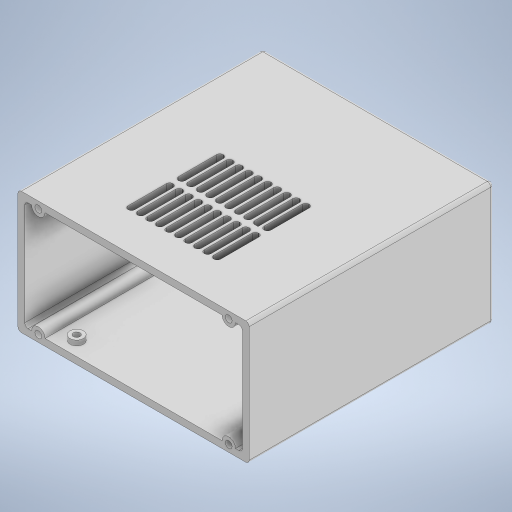
# Autodesk Inventor part: Case_Front
Saved by Autodesk Inventor 2023 (Build 270158000, 158)
## iProperties
Created: 2022-12-05
Part Number: Case_Front
Material: Generic
Document SubType Name: Modeling
Designer: elect
Density: 1 g/cm^3
Appearance: Default
Author: elect
Autodesk Inventor part; units mm, degrees
ref_plane "YZ Plane" through (0, 0, 0) normal (1, 0, 0) x (0, 1, 0)
ref_plane "XZ Plane" through (0, 0, 0) normal (0, 1, 0) x (-1, 0, 0)
ref_plane "XY Plane" through (0, 0, 0) normal (0, 0, 1) x (1, 0, 0)
sketch "Sketch1" plane through (0, 0, 0) normal (0, 0, 1) x (1, 0, 0)
  line L0 (1.5875, 0) -> (106.3625, 0)
  line L1 (107.95, 1.5875) -> (107.95, 55.5625)
  line L2 (106.3625, 57.15) -> (1.5875, 57.15)
  line L3 (0, 55.5625) -> (0, 1.5875)
  arc A0 (1.5875, 57.15) -> (0, 55.5625) centre (1.5875, 55.5625) ccw
  arc A1 (107.95, 55.5625) -> (106.3625, 57.15) centre (106.3625, 55.5625) ccw
  arc A2 (106.3625, 0) -> (107.95, 1.5875) centre (106.3625, 1.5875) ccw
  arc A3 (0, 1.5875) -> (1.5875, 0) centre (1.5875, 1.5875) ccw
  point P0 (0, 0)
  point P1 (107.95, 57.15)
  point P2 (0, 57.15)
  dimension "d0" = 107.95
  dimension "d1" = 57.15
  dimension "d2" = 1.5875
  dimension "d3" = 1.5875
  constraints: 8 end point, 8 point on circle, 8 tangent, 6 point on line, 4 centre point, 2 equal radius, 2 parallel, 1 horizontal, 1 perpendicular
  measures "d0" distance of point (107.95, 57.15) point (0, 57.15)
  measures "d1" distance of point (0, 57.15) point (0, 0)
  measures "d2" radius of A0
  measures "d3" radius of A1
extrude "Extrusion1" add sketch "Sketch1" along normal blind 114.3
sketch "Sketch2" plane through (0, 0, 114.3) normal (0, 0, 1) x (1, 0, 0)
  line L0 (104.775, 52.3875) -> (104.775, 4.7625)
  line L1 (3.175, 4.7625) -> (3.175, 52.3875)
  arc A0 (4.7625, 53.975) -> (3.175, 52.3875) centre (4.7625, 52.3875) ccw
  arc A1 (104.775, 52.3875) -> (103.1875, 53.975) centre (103.1875, 52.3875) ccw
  arc A2 (103.1875, 3.175) -> (104.775, 4.7625) centre (103.1875, 4.7625) ccw
  arc A3 (3.175, 4.7625) -> (4.7625, 3.175) centre (4.7625, 4.7625) ccw
  line L2 (106.3625, 57.15) -> (1.5875, 57.15) projected
  line L3 (0, 55.5625) -> (0, 1.5875) projected
  line L4 (1.5875, 0) -> (106.3625, 0) projected
  line L5 (107.95, 1.5875) -> (107.95, 55.5625) projected
  line L6 (4.7625, 53.975) -> (6.35, 53.975)
  line L7 (12.7, 53.975) -> (95.25, 53.975)
  line L8 (101.6, 53.975) -> (103.1875, 53.975)
  line L9 (103.1875, 3.175) -> (101.6, 3.175)
  line L10 (95.25, 3.175) -> (12.7, 3.175)
  line L11 (6.35, 3.175) -> (4.7625, 3.175)
  arc A4 (6.35, 53.975) -> (12.7, 53.975) centre (9.525, 53.975) ccw
  arc A5 (95.25, 53.975) -> (101.6, 53.975) centre (98.425, 53.975) ccw
  arc A6 (12.7, 3.175) -> (6.35, 3.175) centre (9.525, 3.175) ccw
  arc A7 (101.6, 3.175) -> (95.25, 3.175) centre (98.425, 3.175) ccw
  point P0 (0, 0)
  point P1 (100.0125, 53.975)
  point P2 (11.1125, 53.975)
  dimension "d6" = 1.5875
  dimension "d8" = 3.175
  dimension "d10" = 3.175
  dimension "d73" = 3.175
  dimension "d75" = 6.35
  dimension "d76" = 6.35
  dimension "d77" = 6.35
  constraints: 16 end point, 16 point on circle, 16 tangent, 10 parallel, 8 centre point, 6 equal radius, 4 point on line, 3 horizontal, 3 perpendicular, 2 vertical alignment
  measures "d6" radius of A0
  measures "d8" distance between parallel lines of L1 L3
  measures "d10" distance between parallel lines of L5 L0
  measures "d73" distance between parallel lines of L2 L7
  measures "d75" distance from line of L1 A4.centre
  measures "d76" distance from line of L0 A5.centre
  measures "d77" diameter of A4
extrude "Extrusion2" cut sketch "Sketch2" against normal blind 111.125
fillet "Fillet1" radius 1.5875 8 edges at (0.465, 56.685, 0) (0, 28.575, 0) (0.465, 0.465, 0) (53.975, 0, 0) (107.485, 0.465, 0) (107.95, 28.575, 0) (107.485, 56.685, 0) (53.975, 57.15, 0)
sketch "Sketch3" plane through (0, 0, 0) normal (0, 0, -1) x (-1, 0, 0)
  line L0 (-82.8675, 44.5135) -> (-25.0825, 44.5135)
  line L1 (-23.495, 42.926) -> (-23.495, 20.701)
  line L2 (-25.0825, 19.1135) -> (-82.8675, 19.1135)
  line L3 (-84.455, 20.701) -> (-84.455, 42.926)
  line L4 (-1.5875, 1.5875) -> (-106.3625, 1.5875) projected
  line L5 (-106.3625, 55.5625) -> (-1.5875, 55.5625) projected
  line L6 (-1.5875, 55.5625) -> (-1.5875, 1.5875) projected
  line L7 (-106.3625, 1.5875) -> (-106.3625, 55.5625) projected
  arc A0 (-82.8675, 44.5135) -> (-84.455, 42.926) centre (-82.8675, 42.926) ccw
  arc A1 (-84.455, 20.701) -> (-82.8675, 19.1135) centre (-82.8675, 20.701) ccw
  arc A2 (-25.0825, 19.1135) -> (-23.495, 20.701) centre (-25.0825, 20.701) ccw
  arc A3 (-23.495, 42.926) -> (-25.0825, 44.5135) centre (-25.0825, 42.926) ccw
  point P0 (0, 0)
  point P1 (-84.455, 44.5135)
  point P2 (-23.495, 44.5135)
  point P3 (-84.455, 19.1135)
  point P4 (-23.495, 31.8135)
  dimension "d17" = 60.96
  dimension "d18" = 25.4
  dimension "d19" = 17.526
  dimension "d20" = 11.049
  dimension "d21" = 21.9075
  dimension "d22" = 21.9075
  dimension "d23" = 1.5875
  constraints: 8 end point, 8 point on circle, 8 tangent, 6 point on line, 4 centre point, 3 equal radius, 2 parallel, 1 horizontal, 1 midpoint, 1 perpendicular
  measures "d17" distance of point (-84.455, 44.513) point (-23.495, 44.514)
  measures "d18" distance of point (-84.455, 19.113) point (-84.455, 44.513)
  measures "d19" distance between parallel lines of L4 L2
  measures "d20" distance between parallel lines of L5 L0
  measures "d21" distance from line of L6 point (-23.495, 31.814)
  measures "d22" distance between parallel lines of L7 L3
  measures "d23" radius of A0
extrude "Extrusion3" cut sketch "Sketch3" against normal blind 111.125 contours L0 A3 L1 A2 L2 A1 L3 A0
fillet "Fillet2" radius 1.5875 8 edges at (23.96, 44.0485, 0) (23.495, 31.8135, 0) (23.96, 19.5785, 0) (53.975, 19.1135, 0) (83.99, 19.5785, 0) (84.455, 31.8135, 0) (83.99, 44.0485, 0) (53.975, 44.5135, 0)
sketch "Sketch4" plane through (0, 0, 3.175) normal (0, 0, 1) x (1, 0, 0)
  line L0 (20.955, 47.6885) -> (86.995, 47.6885)
  line L1 (86.995, 47.6885) -> (86.995, 15.9385)
  line L2 (86.995, 15.9385) -> (20.955, 15.9385)
  line L3 (20.955, 15.9385) -> (20.955, 47.6885)
  line L4 (25.0825, 19.1135) -> (82.8675, 19.1135) projected
  line L5 (82.8675, 44.5135) -> (25.0825, 44.5135) projected
  line L6 (23.495, 42.926) -> (23.495, 20.701) projected
  line L7 (84.455, 20.701) -> (84.455, 42.926) projected
  line L8 (43.815, 47.6885) -> (64.135, 47.6885)
  line L9 (64.135, 47.6885) -> (64.135, 50.2285)
  line L10 (64.135, 50.2285) -> (43.815, 50.2285)
  line L11 (43.815, 50.2285) -> (43.815, 47.6885)
  line L12 (86.995, 40.0685) -> (89.535, 40.0685)
  line L13 (89.535, 40.0685) -> (89.535, 23.5585)
  line L14 (89.535, 23.5585) -> (86.995, 23.5585)
  line L15 (86.995, 23.5585) -> (86.995, 40.0685)
  line L16 (43.815, 15.9385) -> (64.135, 15.9385)
  line L17 (64.135, 15.9385) -> (64.135, 13.3985)
  line L18 (64.135, 13.3985) -> (43.815, 13.3985)
  line L19 (43.815, 13.3985) -> (43.815, 15.9385)
  line L20 (20.955, 40.0685) -> (18.415, 40.0685)
  line L21 (18.415, 40.0685) -> (18.415, 23.5585)
  line L22 (18.415, 23.5585) -> (20.955, 23.5585)
  line L23 (20.955, 23.5585) -> (20.955, 40.0685)
  circle A0 centre (12.7, 44.5135) radius 2.54
  circle A1 centre (94.5614, 44.5135) radius 2.54
  circle A2 centre (12.446, 37.1519) radius 2.667
  circle A3 centre (12.446, 28.1095) radius 2.667
  circle A4 centre (12.446, 19.0671) radius 2.667
  circle A5 centre (94.361, 37.1502) radius 2.667
  circle A6 centre (94.361, 28.1078) radius 2.667
  circle A7 centre (94.361, 19.0654) radius 1.5875
  point P0 (0, 0)
  point P1 (19.685, 40.0685)
  point P2 (19.685, 23.5585)
  point P3 (43.815, 48.9585)
  point P4 (64.135, 15.9385)
  point P5 (64.135, 47.6885)
  dimension "d27" = 66.04
  dimension "d28" = 31.75
  dimension "d29" = 3.175
  dimension "d30" = 3.175
  dimension "d31" = 2.54
  dimension "d32" = 2.54
  dimension "d33" = 7.62
  dimension "d34" = 7.62
  dimension "d35" = 2.54
  dimension "d36" = 7.62
  dimension "d37" = 7.62
  dimension "d38" = 2.54
  dimension "d39" = 22.86
  dimension "d40" = 22.86
  dimension "d41" = 2.54
  dimension "d42" = 22.86
  dimension "d43" = 22.86
  dimension "d44" = 2.54
  dimension "d47" = 81.8614
  dimension "d48" = 0
  dimension "d49" = 10.795
  dimension "d50" = 5.08
  dimension "d78" = 5.334
  dimension "d79" = 7.366
  dimension "d80" = 7.366
  dimension "d81" = 9.0424
  dimension "d82" = 9.0424
  dimension "d83" = 9.0424
  dimension "d84" = 9.0424
  dimension "d87" = 3.175
  dimension "d104" = 11.049
  dimension "d105" = 9.906
  constraints: 40 end point, 10 parallel, 8 centre point, 5 equal radius, 5 horizontal, 5 perpendicular, 4 point on line, 4 vertical alignment, 3 midpoint, 1 horizontal alignment
  measures "d27" distance of L0.start L0.end
  measures "d28" distance of L2.end L0.start
  measures "d29" distance between parallel lines of L4 L2
  measures "d30" distance between parallel lines of L5 L0
  measures "d31" distance between parallel lines of L6 L3
  measures "d32" distance between parallel lines of L1 L7
  measures "d33" distance from line of point (19.685, 40.069) L0
  measures "d34" distance from line of L2 point (19.685, 23.558)
  measures "d35" distance between parallel lines of L3 L21
  measures "d36" distance between parallel lines of L2 L14
  measures "d37" distance between parallel lines of L0 L12
  measures "d38" distance between parallel lines of L1 L13
  measures "d39" distance between parallel lines of L1 L9
  measures "d40" distance from line of L3 point (43.815, 48.958)
  measures "d41" distance between parallel lines of L8 L10
  measures "d42" distance between parallel lines of L1 L17
  measures "d43" distance between parallel lines of L3 L19
  measures "d44" distance between parallel lines of L16 L18
  measures "d47" distance of A1.centre A0.centre
  measures "d48" distance from line of L5 A0.centre
  measures "d49" distance from line of L6 A0.centre
  measures "d50" diameter of A0
  measures "d78" diameter of A2
  measures "d79" distance of A0.centre A2.centre
  measures "d80" distance of A1.centre A5.centre
  measures "d81" distance of A3.centre A2.centre
  measures "d82" distance of A4.centre A3.centre
  measures "d83" distance of A6.centre A5.centre
  measures "d84" distance of A6.centre A7.centre
  measures "d87" diameter of A7
  measures "d104" distance from line of L6 A2.centre
  measures "d105" distance from line of L7 A5.centre
extrude "Extrusion4" add sketch "Sketch4" along normal blind 3.175 contours L11 L10 L9 L0 | L3 L22 L21 L20 | L12 L13 L14 L1 | L2 L17 L18 L19
extrude "Extrusion5" cut sketch "Sketch4" against normal blind 25.4 contours A2 | A3 | A4 | A5 | A6 | A7
extrude "Extrusion6" add sketch "Sketch4" along normal blind 12.7 contours A0 | A1
hole "Hole4" at (12.7, 44.5135, 3.175) at (94.5614, 44.5135, 3.175) direction (0, 0, 1) diameter 3.175 end through all
hole "Hole5" at (9.525, 53.975, 114.3) at (98.425, 53.975, 114.3) at (98.425, 3.175, 114.3) at (9.525, 3.175, 114.3) direction (0, 0, -1) diameter 3.175 depth 50.8 tip angle 118
sketch "Sketch5" plane through (12.7, 3.175, 114.3) normal (0, 1, 0) x (1, 0, 0)
  circle A0 centre (8.128, 6.604) radius 3.175
  line L0 (-11.1125, 0) -> (93.6625, 0) projected
  line L1 (-12.7, 112.7125) -> (-12.7, 0) projected
  point P0 (-12.7, 114.3)
  dimension "d106" = 6.35
  dimension "d107" = 6.604
  dimension "d108" = 20.828
  constraints: 1 centre point
  measures "d106" diameter of A0
  measures "d107" distance from line of L0 A0.centre
  measures "d108" distance from line of L1 A0.centre
extrude "Extrusion7" add sketch "Sketch5" along normal blind 2.286
sketch "Sketch6" plane through (20.828, 5.461, 107.696) normal (0, 1, 0) x (1, 0, 0)
  circle A0 centre (0, 0) radius 3.175 projected
  point P0 (-20.828, 107.696)
  constraints: 1 coincident
hole "Hole6" at (20.828, 5.461, 107.696) direction (0, -1, 0) diameter 3.175 depth 3.175 tip angle 118
sketch "Sketch7" plane through (0, 0, 0) normal (0, 0, -1) x (-1, 0, 0)
  line L0 (-84.7724, 13.1636) -> (-21.2726, 13.0175) construction
  line L1 (-21.2726, 13.0175) -> (-21.3018, 0.3175) construction
  line L2 (-21.3018, 0.3175) -> (-84.8016, 0.4636) construction
  line L3 (-84.8016, 0.4636) -> (-84.7724, 13.1636) construction
  line L4 (-106.3625, 1.5875) -> (-106.3625, 55.5625) projected
  line L5 (-1.5875, 1.5875) -> (-106.3625, 1.5875) projected
  line L6 (-106.3625, 55.5625) -> (-1.5875, 55.5625)
  line L7 (-1.5875, 55.5625) -> (-1.5875, 1.5875)
  line L8 (-100.711, 43.307) -> (-88.011, 43.307) construction
  line L9 (-88.011, 43.307) -> (-88.011, 40.132) construction
  line L10 (-88.011, 40.132) -> (-100.711, 40.132) construction
  line L11 (-100.711, 40.132) -> (-100.711, 43.307) construction
  line L12 (-100.711, 34.163) -> (-88.011, 34.163) construction
  line L13 (-88.011, 34.163) -> (-88.011, 30.988) construction
  line L14 (-88.011, 30.988) -> (-100.711, 30.988) construction
  line L15 (-100.711, 30.988) -> (-100.711, 34.163) construction
  line L16 (-100.711, 25.273) -> (-88.011, 25.273) construction
  line L17 (-88.011, 25.273) -> (-88.011, 22.098) construction
  line L18 (-88.011, 22.098) -> (-100.711, 22.098) construction
  line L19 (-100.711, 22.098) -> (-100.711, 25.273) construction
  line L20 (-82.8675, 17.526) -> (-25.0825, 17.526) projected
  circle A0 centre (-94.361, 37.1502) radius 2.667 projected
  line L21 (-21.336, 43.307) -> (-3.556, 43.307) construction
  line L22 (-3.556, 43.307) -> (-3.556, 40.132) construction
  line L23 (-3.556, 40.132) -> (-21.336, 40.132) construction
  line L24 (-21.336, 40.132) -> (-21.336, 43.307) construction
  line L25 (-21.336, 34.163) -> (-3.556, 34.163) construction
  line L26 (-3.556, 34.163) -> (-3.556, 30.988) construction
  line L27 (-3.556, 30.988) -> (-21.336, 30.988) construction
  line L28 (-21.336, 30.988) -> (-21.336, 34.163) construction
  line L29 (-21.336, 25.273) -> (-3.556, 25.273) construction
  line L30 (-3.556, 25.273) -> (-3.556, 22.098) construction
  line L31 (-3.556, 22.098) -> (-21.336, 22.098) construction
  line L32 (-21.336, 22.098) -> (-21.336, 25.273) construction
  circle A1 centre (-12.446, 37.1519) radius 2.667 projected
  line L33 (-59.3387, 12.9994) -> (-57.4495, 12.9951)
  line L34 (-57.4495, 12.9951) -> (-57.4571, 9.6802)
  spline S0 degree 2 poles (-57.4571, 9.6802) (-57.4595, 8.6417) (-57.8317, 7.5512) (-58.954, 6.7969) (-59.8224, 6.7989) knots 0 0 0 1 2 3 3 3
  spline S1 degree 2 poles (-59.8224, 6.7989) (-60.7435, 6.8011) (-61.7574, 7.3021) (-62.3067, 8.2656) (-62.3579, 8.9698) knots 0 0 0 1 2 3 3 3
  line L35 (-62.3579, 8.9698) -> (-60.5561, 9.212)
  spline S2 degree 2 poles (-60.5561, 9.212) (-60.5512, 8.8072) (-60.423, 8.4197) (-60.2648, 8.2961) knots 0 0 0 1 2 2 2
  spline S3 degree 2 poles (-60.2648, 8.2961) (-60.1594, 8.2196) (-59.9599, 8.2191) knots 0 0 0 1 1 1
  spline S4 degree 2 poles (-59.9599, 8.2191) (-59.6431, 8.2184) (-59.3487, 8.6871) (-59.3474, 9.2445) knots 0 0 0 1 2 2 2
  line L36 (-59.3474, 9.2445) -> (-59.3387, 12.9994)
  line L37 (-56.1587, 12.9921) -> (-53.3601, 12.9857)
  spline S5 degree 2 poles (-53.3601, 12.9857) (-52.5328, 12.9838) (-51.513, 12.5297) (-50.8519, 11.6891) (-50.5553, 10.5737) (-50.5567, 9.9518) knots 0 0 0 1 2 3 4 4 4
  spline S6 degree 2 poles (-50.5567, 9.9518) (-50.559, 8.972) (-51.0073, 7.8993) (-51.7952, 7.1736) (-52.2531, 7.0514) knots 0 0 0 1 2 3 3 3
  spline S7 degree 2 poles (-52.2531, 7.0514) (-52.8696, 6.8885) (-53.3741, 6.8897) knots 0 0 0 1 1 1
  line L38 (-53.3741, 6.8897) -> (-56.1728, 6.8961)
  line L39 (-56.1728, 6.8961) -> (-56.1587, 12.9921)
  line L40 (-54.2786, 11.609) -> (-54.2862, 8.2765)
  line L41 (-54.2862, 8.2765) -> (-53.8227, 8.2754)
  spline S8 degree 2 poles (-53.8227, 8.2754) (-53.236, 8.2741) (-52.7367, 8.5369) (-52.4536, 9.1875) (-52.4519, 9.9209) knots 0 0 0 1 2 3 3 3
  spline S9 degree 2 poles (-52.4519, 9.9209) (-52.4496, 10.889) (-53.0817, 11.6063) (-53.8092, 11.6079) knots 0 0 0 1 2 2 2
  line L42 (-53.8092, 11.6079) -> (-54.2786, 11.609)
  line L43 (-45.5064, 9.3652) -> (-43.8589, 8.8627)
  spline S10 degree 2 poles (-43.8589, 8.8627) (-44.0247, 8.1707) (-44.7427, 7.2395) (-45.8057, 6.7667) (-46.6213, 6.7686) knots 0 0 0 1 2 3 3 3
  spline S11 degree 2 poles (-46.6213, 6.7686) (-47.6187, 6.7709) (-48.8729, 7.3546) (-49.7849, 8.8118) (-49.7822, 9.9441) knots 0 0 0 1 2 3 3 3
  spline S12 degree 2 poles (-49.7822, 9.9441) (-49.7788, 11.4579) (-48.1674, 13.0794) (-46.6948, 13.076) knots 0 0 0 1 2 2 2
  spline S13 degree 2 poles (-46.6948, 13.076) (-45.5448, 13.0733) (-44.2327, 12.1374) (-43.9122, 11.1745) knots 0 0 0 1 2 2 2
  line L44 (-43.9122, 11.1745) -> (-45.5793, 10.8087)
  spline S14 degree 2 poles (-45.5793, 10.8087) (-45.6667, 11.0846) (-45.7603, 11.2139) knots 0 0 0 1 1 1
  spline S15 degree 2 poles (-45.7603, 11.2139) (-45.9182, 11.4314) (-46.3753, 11.6671) (-46.6569, 11.6678) knots 0 0 0 1 2 2 2
  spline S16 degree 2 poles (-46.6569, 11.6678) (-47.2906, 11.6692) (-47.6321, 11.1537) knots 0 0 0 1 1 1
  spline S17 degree 2 poles (-47.6321, 11.1537) (-47.8911, 10.7729) (-47.893, 9.9515) knots 0 0 0 1 1 1
  spline S18 degree 2 poles (-47.893, 9.9515) (-47.8953, 8.9365) (-47.281, 8.1841) (-46.7236, 8.1828) knots 0 0 0 1 2 2 2
  spline S19 degree 2 poles (-46.7236, 8.1828) (-46.1838, 8.1816) (-45.6309, 8.7846) (-45.5064, 9.3652) knots 0 0 0 1 2 2 2
  point P0 (0, 0)
  point P1 (-53.0225, 13.0905)
  point P2 (-21.2872, 6.6675)
  point P3 (-94.361, 43.307)
  point P4 (-94.361, 34.163)
  point P5 (-94.361, 25.273)
  point P6 (-100.711, 23.6855)
  point P7 (-12.446, 43.307)
  point P8 (-12.446, 34.163)
  point P9 (-12.446, 25.273)
  point P10 (-88.011, 41.7195)
  point P11 (-21.336, 41.7195)
  point P12 (-21.336, 32.5755)
  point P13 (-88.011, 32.5755)
  point P14 (-88.011, 23.6855)
  point P15 (-21.336, 23.6855)
  dimension "d118" = 53.34
  dimension "d119" = 5.08
  dimension "d120" = 12.7
  dimension "d121" = 63.5
  dimension "d124" = 12.7
  dimension "d125" = 12.7
  dimension "d126" = 12.7
  dimension "d127" = 3.175
  dimension "d128" = 3.175
  dimension "d129" = 3.175
  dimension "d134" = 17.78
  dimension "d135" = 17.78
  dimension "d136" = 17.78
  dimension "d137" = 3.175
  dimension "d138" = 3.175
  dimension "d139" = 3.175
  dimension "d140" = 4.572
  dimension "d141" = 13.462
  dimension "d142" = 22.606
  constraints: 15 midpoint, 6 vertical alignment, 4 end point, 3 horizontal alignment, 2 coincident, 1 horizontal, 1 perpendicular, 14 other
  measures "d118" distance from line of L4 point (-53.022, 13.091)
  measures "d119" distance from line of L5 point (-21.287, 6.668)
  measures "d120" distance between parallel lines of L2 L0
  measures "d121" distance of L0.start L0.end
  measures "d124" distance of L16.start L16.end
  measures "d125" distance of L12.start L12.end
  measures "d126" distance of L8.start L8.end
  measures "d127" distance of L8.end L9.end
  measures "d128" distance of L12.end L13.end
  measures "d129" distance of L16.end L17.end
  measures "d134" distance of L21.start L21.end
  measures "d135" distance of L25.start L25.end
  measures "d136" distance of L29.start L29.end
  measures "d137" distance of L21.end L22.end
  measures "d138" distance of L25.end L26.end
  measures "d139" distance of L29.end L30.end
  measures "d140" distance between parallel lines of L20 L31
  measures "d141" distance between parallel lines of L20 L27
  measures "d142" distance between parallel lines of L20 L23
sketch "Sketch8" plane through (1.5875, 57.15, 114.3) normal (0, 1, 0) x (1, 0, 0)
  line L0 (30.7975, 61.9125) -> (33.9725, 61.9125)
  line L1 (33.9725, 61.9125) -> (33.9725, 17.4625)
  line L2 (33.9725, 17.4625) -> (30.7975, 17.4625)
  line L3 (30.7975, 17.4625) -> (30.7975, 61.9125)
  line L4 (0, 112.7125) -> (0, 0) projected
  line L5 (0, 103.6948) -> (98.6325, 103.6948)
  line L6 (100.0125, 0) -> (100.0125, 111.125) projected
  line L7 (38.4175, 61.9125) -> (38.4175, 17.4625)
  line L8 (35.2425, 17.4625) -> (35.2425, 61.9125)
  line L9 (35.2425, 61.9125) -> (38.4175, 61.9125)
  line L10 (38.4175, 17.4625) -> (35.2425, 17.4625)
  line L11 (42.8625, 61.9125) -> (42.8625, 17.4625)
  line L12 (39.6875, 17.4625) -> (39.6875, 61.9125)
  line L13 (39.6875, 61.9125) -> (42.8625, 61.9125)
  line L14 (42.8625, 17.4625) -> (39.6875, 17.4625)
  line L15 (47.3075, 61.9125) -> (47.3075, 17.4625)
  line L16 (44.1325, 17.4625) -> (44.1325, 61.9125)
  line L17 (44.1325, 61.9125) -> (47.3075, 61.9125)
  line L18 (47.3075, 17.4625) -> (44.1325, 17.4625)
  line L19 (51.7525, 61.9125) -> (51.7525, 17.4625)
  line L20 (48.5775, 17.4625) -> (48.5775, 61.9125)
  line L21 (48.5775, 61.9125) -> (51.7525, 61.9125)
  line L22 (51.7525, 17.4625) -> (48.5775, 17.4625)
  line L23 (56.1975, 61.9125) -> (56.1975, 17.4625)
  line L24 (53.0225, 17.4625) -> (53.0225, 61.9125)
  line L25 (53.0225, 61.9125) -> (56.1975, 61.9125)
  line L26 (56.1975, 17.4625) -> (53.0225, 17.4625)
  line L27 (60.6425, 61.9125) -> (60.6425, 17.4625)
  line L28 (57.4675, 17.4625) -> (57.4675, 61.9125)
  line L29 (57.4675, 61.9125) -> (60.6425, 61.9125)
  line L30 (60.6425, 17.4625) -> (57.4675, 17.4625)
  line L31 (65.0875, 61.9125) -> (65.0875, 17.4625)
  line L32 (61.9125, 17.4625) -> (61.9125, 61.9125)
  line L33 (61.9125, 61.9125) -> (65.0875, 61.9125)
  line L34 (65.0875, 17.4625) -> (61.9125, 17.4625)
  line L35 (69.5325, 61.9125) -> (69.5325, 17.4625)
  line L36 (66.3575, 17.4625) -> (66.3575, 61.9125)
  line L37 (66.3575, 61.9125) -> (69.5325, 61.9125)
  line L38 (69.5325, 17.4625) -> (66.3575, 17.4625)
  line L39 (73.9775, 61.9125) -> (73.9775, 17.4625)
  line L40 (70.8025, 17.4625) -> (70.8025, 61.9125)
  line L41 (70.8025, 61.9125) -> (73.9775, 61.9125)
  line L42 (73.9775, 17.4625) -> (70.8025, 17.4625)
  line L43 (104.775, 112.7125) -> (104.775, 0) projected
  line L44 (0, 112.7125) -> (104.775, 112.7125) projected
  line L45 (30.7975, 40.9575) -> (33.9725, 40.9575)
  line L46 (30.7975, 38.4175) -> (33.9725, 38.4175)
  line L47 (35.2425, 38.4175) -> (38.4175, 38.4175)
  line L48 (35.2425, 40.9575) -> (38.4175, 40.9575)
  line L49 (39.6875, 40.9575) -> (42.8625, 40.9575)
  line L50 (39.6875, 38.4175) -> (42.8625, 38.4175)
  line L51 (44.1325, 40.9575) -> (47.3075, 40.9575)
  line L52 (44.1325, 38.4175) -> (47.3075, 38.4175)
  line L53 (48.5775, 40.9575) -> (51.7525, 40.9575)
  line L54 (48.5775, 38.4175) -> (51.7525, 38.4175)
  line L55 (53.0225, 40.9575) -> (56.1975, 40.9575)
  line L56 (53.0225, 38.4175) -> (56.1975, 38.4175)
  line L57 (57.4675, 40.9575) -> (60.6425, 40.9575)
  line L58 (57.4675, 38.4175) -> (60.6425, 38.4175)
  line L59 (61.9125, 40.9575) -> (65.0875, 40.9575)
  line L60 (61.9125, 38.4175) -> (65.0875, 38.4175)
  line L61 (66.3575, 40.9575) -> (69.5325, 40.9575)
  line L62 (70.8025, 40.9575) -> (73.9775, 40.9575)
  line L63 (66.3575, 38.4175) -> (69.5325, 38.4175)
  line L64 (70.8025, 38.4175) -> (73.9775, 38.4175)
  line L65 (30.7975, 40.9575) -> (30.7975, 38.4175)
  line L66 (33.9725, 38.4175) -> (33.9725, 40.9575)
  line L67 (35.2425, 40.9575) -> (35.2425, 38.4175)
  line L68 (38.4175, 40.9575) -> (38.4175, 38.4175)
  line L69 (39.6875, 40.9575) -> (39.6875, 38.4175)
  line L70 (42.8625, 40.9575) -> (42.8625, 38.4175)
  line L71 (44.1325, 40.9575) -> (44.1325, 38.4175)
  line L72 (47.3075, 38.4175) -> (47.3075, 40.9575)
  line L73 (48.5775, 40.9575) -> (48.5775, 38.4175)
  line L74 (51.7525, 40.9575) -> (51.7525, 38.4175)
  line L75 (53.0225, 40.9575) -> (53.0225, 38.4175)
  line L76 (56.1975, 40.9575) -> (56.1975, 38.4175)
  line L77 (57.4675, 40.9575) -> (57.4675, 38.4175)
  line L78 (60.6425, 40.9575) -> (60.6425, 38.4175)
  line L79 (61.9125, 40.9575) -> (61.9125, 38.4175)
  line L80 (65.0875, 40.9575) -> (65.0875, 38.4175)
  line L81 (66.3575, 38.4175) -> (66.3575, 40.9575)
  line L82 (69.5325, 40.9575) -> (69.5325, 38.4175)
  line L83 (70.8025, 40.9575) -> (70.8025, 38.4175)
  line L84 (73.9775, 40.9575) -> (73.9775, 38.4175)
  point P0 (-1.5875, 114.3)
  dimension "d143" = 3.175
  dimension "d144" = 44.45
  dimension "d147" = 4.445
  dimension "d152" = 30.7975
  dimension "d153" = 30.7975
  dimension "d154" = 50.8
  constraints: 162 end point, 41 point on line, 25 perpendicular, 14 collinear, 5 parallel, 2 horizontal, 72 other
  measures "d143" distance of L1.end L2.end
  measures "d144" distance of L2.end L0.start
  measures "d147" distance of L0.end L7.start
  measures "d152" distance between parallel lines of L4 L3
  measures "d153" distance between parallel lines of L43 L39
  measures "d154" distance between parallel lines of L0 L44
extrude "Extrusion8" cut sketch "Sketch8" against normal blind 25.4 contours L0 L1 L45 L3 | L46 L1 L2 L3 | L7 L48 L8 L9 | L7 L10 L8 L47 | L11 L49 L12 L13 | L11 L14 L12 L50 | L15 L51 L16 L17 | L15 L18 L16 L52 | L19 L53 L20 L21 | L19 L22 L20 L54 | L23 L55 L24 L25 | L23 L26 L24 L56 | L27 L57 L28 L29 | L27 L30 L28 L58 | L31 L59 L32 L33 | L31 L34 L32 L60 | L35 L61 L36 L37 | L35 L38 L36 L63 | L39 L62 L40 L41 | L39 L42 L40 L64
sketch "Sketch9" plane through (12.7, 53.975, 114.3) normal (0, -1, 0) x (1, 0, 0)
  line L0 (14.2875, -63.7812) -> (68.2625, -63.7812)
  line L1 (68.2625, -63.7812) -> (68.2625, -66.9562)
  line L2 (68.2625, -66.9562) -> (14.2875, -66.9562)
  line L3 (14.2875, -66.9562) -> (14.2875, -63.7812)
  line L4 (68.2625, -63.7812) -> (65.0875, -63.7812)
  line L5 (65.0875, -63.7812) -> (65.0875, -12.9812)
  line L6 (65.0875, -12.9812) -> (68.2625, -12.9812)
  line L7 (68.2625, -12.9812) -> (68.2625, -63.7812)
  line L8 (19.685, -17.4625) -> (19.685, -61.9125) projected
  line L9 (14.2875, -63.7812) -> (17.4625, -63.7812)
  line L10 (17.4625, -63.7812) -> (17.4625, -12.9812)
  line L11 (17.4625, -12.9812) -> (14.2875, -12.9812)
  line L12 (14.2875, -12.9812) -> (14.2875, -63.7812)
  line L13 (62.865, -61.9125) -> (62.865, -17.4625) projected
  point P0 (-12.7, -114.3)
  dimension "d157" = 53.975
  dimension "d158" = 3.175
  dimension "d159" = 3.175
  dimension "d160" = 5.3975
  dimension "d161" = 50.8
  dimension "d162" = 50.8
  dimension "d163" = 3.175
  dimension "d164" = 5.3975
  dimension "d165" = 47.625
  constraints: 24 end point, 6 parallel, 3 horizontal, 3 perpendicular
  measures "d157" distance of L1.end L2.end
  measures "d158" distance of L0.end L1.end
  measures "d159" distance between parallel lines of L7 L5
  measures "d160" distance between parallel lines of L8 L3
  measures "d161" distance of L11.end L0.start
  measures "d162" distance of L6.end L0.end
  measures "d163" distance between parallel lines of L10 L12
  measures "d164" distance between parallel lines of L13 L7
  measures "d165" distance between parallel lines of L5 L10
extrude "Extrusion9" add sketch "Sketch9" along normal blind 3.175
sketch "Sketch10" plane through (12.7, 50.8, 114.3) normal (0, -1, 0) x (1, 0, 0)
  line L0 (14.2875, -66.9562) -> (14.2875, -12.9812) projected
  line L1 (68.2625, -66.9562) -> (14.2875, -66.9562) projected
  line L2 (14.2875, -12.9812) -> (20.6375, -12.9812)
  line L3 (20.6375, -12.9812) -> (20.6375, -66.9562)
  line L4 (20.6375, -66.9562) -> (14.2875, -66.9562)
  line L5 (14.2875, -66.9562) -> (14.2875, -12.9812)
  line L6 (68.2625, -12.9812) -> (61.9125, -12.9812)
  line L7 (61.9125, -12.9812) -> (61.9125, -66.9562)
  line L8 (61.9125, -66.9562) -> (68.2625, -66.9562)
  line L9 (68.2625, -66.9562) -> (68.2625, -12.9812)
  line L10 (68.2625, -12.9812) -> (68.2625, -66.9562) projected
  line L11 (20.6375, -66.9562) -> (61.9125, -66.9562)
  line L12 (61.9125, -66.9562) -> (61.9125, -60.6062)
  line L13 (61.9125, -60.6062) -> (20.6375, -60.6062)
  line L14 (20.6375, -60.6062) -> (20.6375, -66.9562)
  point P0 (-12.7, -114.3)
  point P1 (41.275, -66.9562)
  point P2 (20.6375, -60.6062)
  dimension "d168" = 6.35
  dimension "d169" = 6.35
  dimension "d170" = 0
  dimension "d171" = 6.35
  constraints: 24 end point, 6 parallel, 4 point on line, 3 horizontal, 3 perpendicular, 1 midpoint
  measures "d168" distance of L0.end L2.end
  measures "d169" distance of L6.start L6.end
  measures "d170" distance between parallel lines of L10 L9
  measures "d171" distance from line of point (41.275, -66.956) L13
extrude "Extrusion10" add sketch "Sketch10" along normal blind 1.5875
chamfer "Chamfer2" distance 3.81 angle 50 1 edges at (53.975, 49.2125, 47.3438) measured on face at (53.975, 49.2125, 47.8438)
fillet "Fillet3" radius 3.175 2 edges at (26.9875, 49.2125, 76.2363) (80.9625, 49.2125, 76.2363)
fillet "Fillet4" radius 1.524 79 edges at (32.385, 55.5625, 52.3875) (36.83, 55.5625, 52.3875) (41.275, 55.5625, 52.3875) (45.72, 55.5625, 52.3875) (50.165, 55.5625, 52.3875) (54.61, 55.5625, 52.3875) (59.055, 55.5625, 52.3875) (63.5, 55.5625, 52.3875) (67.945, 55.5625, 52.3875) (72.39, 55.5625, 52.3875) (35.56, 55.5625, 52.3875) (40.005, 55.5625, 52.3875) (44.45, 55.5625, 52.3875) (48.895, 55.5625, 52.3875) (53.34, 55.5625, 52.3875) (57.785, 55.5625, 52.3875) (62.23, 55.5625, 52.3875) (66.675, 55.5625, 52.3875) (71.12, 55.5625, 52.3875) (75.565, 55.5625, 52.3875) (32.385, 55.5625, 96.8375) (36.83, 55.5625, 96.8375) (41.275, 55.5625, 96.8375) (45.72, 55.5625, 96.8375) (50.165, 55.5625, 96.8375) (54.61, 55.5625, 96.8375) (59.055, 55.5625, 96.8375) (63.5, 55.5625, 96.8375) (67.945, 55.5625, 96.8375) (72.39, 55.5625, 96.8375) (75.565, 55.5625, 96.8375) (71.12, 55.5625, 96.8375) (66.675, 55.5625, 96.8375) (62.23, 55.5625, 96.8375) (57.785, 55.5625, 96.8375) (53.34, 55.5625, 96.8375) (48.895, 55.5625, 96.8375) (44.45, 55.5625, 96.8375) (40.005, 55.5625, 96.8375) (35.56, 55.5625, 96.8375) (32.385, 55.5625, 75.8825) (36.83, 55.5625, 75.8825) (41.275, 55.5625, 75.8825) (45.72, 55.5625, 75.8825) (50.165, 55.5625, 75.8825) (54.61, 55.5625, 75.8825) (59.055, 55.5625, 75.8825) (63.5, 55.5625, 75.8825) (67.945, 55.5625, 75.8825) (72.39, 55.5625, 75.8825) (75.565, 55.5625, 75.8825) (71.12, 55.5625, 75.8825) (66.675, 55.5625, 75.8825) (62.23, 55.5625, 75.8825) (57.785, 55.5625, 75.8825) (53.34, 55.5625, 75.8825) (48.895, 55.5625, 75.8825) (44.45, 55.5625, 75.8825) (40.005, 55.5625, 75.8825) (35.56, 55.5625, 75.8825) (32.385, 55.5625, 73.3425) (36.83, 55.5625, 73.3425) (41.275, 55.5625, 73.3425) (45.72, 55.5625, 73.3425) (50.165, 55.5625, 73.3425) (54.61, 55.5625, 73.3425) (59.055, 55.5625, 73.3425) (63.5, 55.5625, 73.3425) (67.945, 55.5625, 73.3425) (72.39, 55.5625, 73.3425) (35.56, 55.5625, 73.3425) (40.005, 55.5625, 73.3425) (44.45, 55.5625, 73.3425) (48.895, 55.5625, 73.3425) (53.34, 55.5625, 73.3425) (57.785, 55.5625, 73.3425) (62.23, 55.5625, 73.3425) (66.675, 55.5625, 73.3425) (75.565, 55.5625, 73.3425)
chamfer "Chamfer3" distance 1.5875 angle 45 1 edges at (92.7735, 19.0654, 0)
emboss "Emboss2" sketch "Sketch7" operation cut depth 1.5875 direction (0, 0, 1) contours L33 L34 S0 S1 L35 S2 S3 S4 L36 | L37 S5 S6 S7 L38 L39 | L43 S10 S11 S12 S13 L44 S14 S15 S16 S17 S18 S19
fillet "Fillet5" radius 1.5875 4 edges at (86.995, 31.8135, 6.35) (53.975, 15.9385, 6.35) (20.955, 31.8135, 6.35) (53.975, 47.6885, 6.35)
fillet "Fillet6" radius 1.5875 6 edges at (91.694, 37.1502, 0) (91.694, 28.1078, 0) (9.779, 37.1519, 0) (9.779, 28.1095, 0) (9.779, 19.0671, 0) (91.186, 19.0654, 0)
fillet "Fillet7" radius 1.5875 3 edges at (33.3375, 50.8, 77.5063) (53.975, 50.8, 53.6938) (74.6125, 50.8, 77.5063)
chamfer "Chamfer4" distance 0.7937 angle 45 5 edges at (9.779, 37.1519, 3.175) (9.779, 28.1095, 3.175) (9.779, 19.0671, 3.175) (91.694, 37.1502, 3.175) (91.694, 28.1078, 3.175)
body "Solid1"
